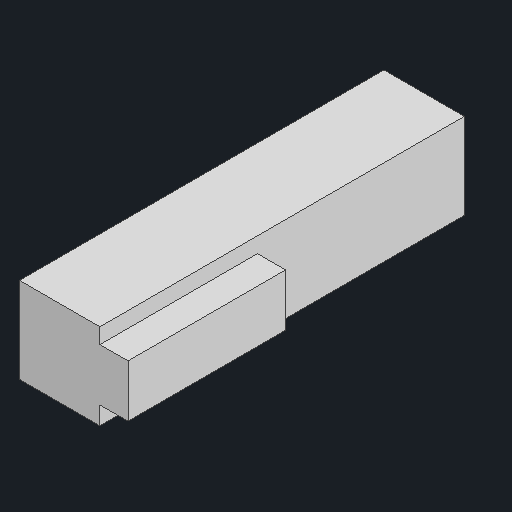
# Autodesk Inventor part: smolLipo
Saved by Autodesk Inventor 2023 (Build 270158000, 158)
## iProperties
Created: 2024-04-13
Part Number: smolLipo
Material: Generic
Document SubType Name: Modeling
Designer: szymo
Density: 1 g/cm^3
Appearance: Default
Mass: 17.824 g
Surface Area: 51.0701 cm^2
Volume: 17.824 cm^3
Author: szymo
Autodesk Inventor part; units mm, degrees
ref_plane "YZ Plane" through (0, 0, 0) normal (1, 0, 0) x (0, 1, 0)
ref_plane "XZ Plane" through (0, 0, 0) normal (0, 1, 0) x (-1, 0, 0)
ref_plane "XY Plane" through (0, 0, 0) normal (0, 0, 1) x (1, 0, 0)
sketch "Sketch1" plane through (0, 0, 0) normal (0, 1, 0) x (-1, 0, 0)
  line L0 (0, 0) -> (-15, 0)
  line L1 (-15, 0) -> (-15, -68)
  line L2 (-15, -68) -> (0, -68)
  line L3 (0, -68) -> (0, 0)
  dimension "d0" = 15
  dimension "d1" = 68
  constraints: 8 end point, 2 parallel, 1 horizontal, 1 perpendicular
  measures "d0" distance of L2.end L1.end
  measures "d1" distance of L1.end L0.end
extrude "Extrusion1" add sketch "Sketch1" along normal blind 16
sketch "Sketch2" plane through (15, 0, 0) normal (1, 0, 0) x (0, 0, -1)
  line L0 (34.4, 3.375) -> (29.4, 3.375) projected
  line L1 (34.4, 13.119) -> (29.4, 13.119) projected
  line L2 (0, 0) -> (0, 16) projected
  line L3 (29.4, 13.119) -> (0, 13.119)
  line L4 (0, 13.119) -> (0, 3.375)
  line L5 (0, 3.375) -> (29.4, 3.375)
  line L6 (29.4, 3.375) -> (29.4, 13.119)
  constraints: 8 end point, 2 parallel, 1 horizontal, 1 perpendicular, 1 point on line
extrude "Extrusion2" add sketch "Sketch2" along normal up to surface (5.25 mm away)
body "Solid1"
